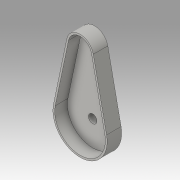
# Autodesk Inventor part: ChainGuard
Saved by Autodesk Inventor 2016 (Build 200138000, 138)
## iProperties
Created: 2017-02-15
Part Number: ChainGuard
Material: Generic
Document SubType Name: Modeling
Designer: Delta
Density: 1 g/cm^3
Appearance: Default
Author: Delta
Autodesk Inventor part; units mm, degrees
ref_plane "YZ Plane" through (0, 0, 0) normal (1, 0, 0) x (0, 1, 0)
ref_plane "XZ Plane" through (0, 0, 0) normal (0, 1, 0) x (-1, 0, 0)
ref_plane "XY Plane" through (0, 0, 0) normal (0, 0, 1) x (1, 0, 0)
sketch "Sketch1" plane through (0, 0, 0) normal (0, 0, 1) x (1, 0, 0)
  arc A0 (-37.287, 7.8288) -> (37.287, 7.8288) centre (0, 0) ccw
  arc A1 (18.6435, 96.6244) -> (-18.6435, 96.6244) centre (0, 92.71) ccw
  line L0 (-18.6435, 96.6244) -> (-37.287, 7.8288)
  line L1 (18.6435, 96.6244) -> (37.287, 7.8288)
  dimension "d0" = 76.2
  dimension "d1" = 38.1
  dimension "d2" = 149.86
  constraints: 4 end point, 4 point on circle, 4 tangent, 2 centre point, 1 coincident
  measures "d0" diameter of A0
  measures "d1" diameter of A1
extrude "Extrusion1" add sketch "Sketch1" along normal blind 20.32
shell "Shell1" thickness 2.54 removed faces 1 at (-6.2145, 37.4273, 20.32)
sketch "Sketch2" plane through (0, 0, 0) normal (0, 0, -1) x (-1, 0, 0)
  circle A0 centre (0, 0) radius 5.969
  arc A1 (-37.287, 7.8288) -> (37.287, 7.8288) centre (0, 0) ccw projected
  circle A2 centre (0, 0) radius 10.795
  dimension "d6" = 11.938
  dimension "d7" = 21.59
  constraints: 2 centre point, 2 coincident
  measures "d6" diameter of A0
  measures "d7" diameter of A2
extrude "Extrusion2" add sketch "Sketch2" along normal blind 7.62
hole "Hole1" at (0, 0, 0) direction (0, 0, 1) diameter 11.938 end through all
body "Solid1"
